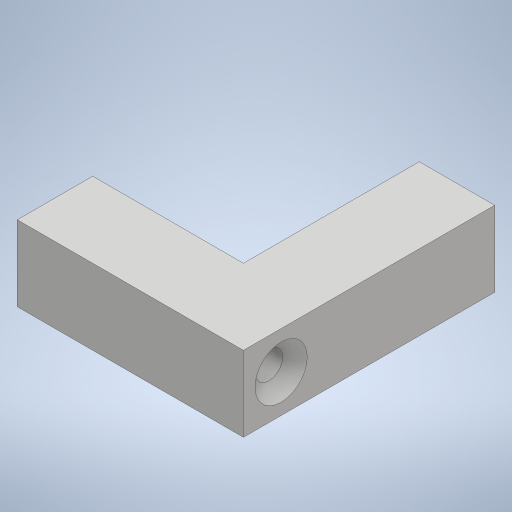
# Autodesk Inventor part: Soporte lamina centelladora
Saved by Autodesk Inventor 2024.2 (Build 282272000, 272)
## iProperties
Created: 2025-06-13
Part Number: Soporte lamina centelladora
Material: Genérico
Document SubType Name: Modeling
Designer: jd.castellanosq
Density: 1 g/cm^3
Appearance: Valor por defecto
Author: jd.castellanosq
Autodesk Inventor part; units mm, degrees
ref_plane "YZ Plane" through (0, 0, 0) normal (1, 0, 0) x (0, 1, 0)
ref_plane "XZ Plane" through (0, 0, 0) normal (0, 1, 0) x (-1, 0, 0)
ref_plane "XY Plane" through (0, 0, 0) normal (0, 0, 1) x (1, 0, 0)
sketch "Boceto1" plane through (0, 0, 0) normal (0, 0, 1) x (1, 0, 0)
  line L0 (0, 0) -> (45, 0)
  line L1 (45, 0) -> (45, 50)
  line L2 (45, 50) -> (30, 50)
  line L3 (30, 50) -> (30, 15)
  line L4 (30, 15) -> (0, 15)
  line L5 (0, 0) -> (0, 15)
  dimension "d0" = 15
  dimension "d1" = 30
  dimension "d2" = 15
  dimension "d3" = 50
  constraints: 12 end point, 4 perpendicular, 1 horizontal, 1 vertical
  measures "d0" distance between parallel lines of L4 L0
  measures "d1" distance between parallel lines of L3 L5
  measures "d2" distance between parallel lines of L1 L3
  measures "d3" distance between parallel lines of L0 L2
extrude "Extrusión1" add sketch "Boceto1" along normal blind 15
sketch "Boceto2" plane through (45, 0, 0) normal (1, 0, 0) x (0, 0, -1)
  line L0 (0, 0) -> (-15, 0) projected
  point P0 (-7.5, 7.5)
  point P1 (-7.5, 0)
  point P2 (-7.5, 0)
  dimension "d6" = 7.5
  constraints: 2 midpoint, 1 vertical alignment
  measures "d6" distance of point (-7.5, 7.5) point (-7.5, 0)
hole "Agujero1" at (45, 7.5, 7.5) direction (-1, 0, 0) diameter 5.5 end through all countersink diameter 10.4 countersink angle 90 clearance for "Tornillo para maquinaria de cabeza plana" size "M5" standard "Perfil M métrico ANSI"
